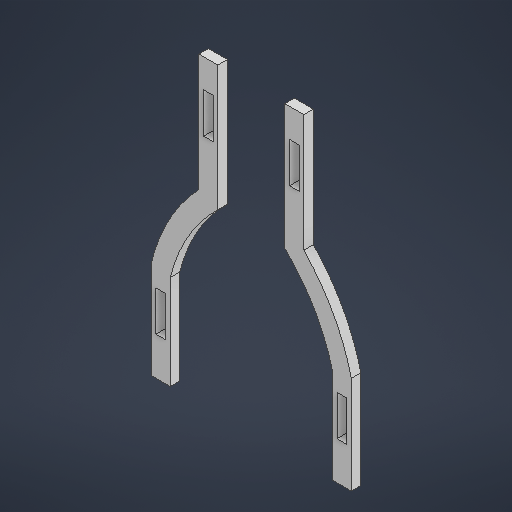
# Autodesk Inventor part: middlelsidewall
Saved by Autodesk Inventor 2026.2 (Build 302298000, 298)
## iProperties
Created: 2026-04-17
Part Number: middlelsidewall
Material: Generic
Document SubType Name: Modeling
Designer: danda
Density: 1 g/cm^3
Appearance: Default
Author: danda
Autodesk Inventor part; units mm, degrees
ref_plane "YZ Plane" through (0, 0, 0) normal (1, 0, 0) x (0, 1, 0)
ref_plane "XZ Plane" through (0, 0, 0) normal (0, 1, 0) x (-1, 0, 0)
ref_plane "XY Plane" through (0, 0, 0) normal (0, 0, 1) x (1, 0, 0)
sketch "Sketch2" plane through (0, 0, 0) normal (0, 0, 1) x (1, 0, 0)
  line L0 (32.8823, 96.9088) -> (32.8823, 36.9088)
  line L1 (-2.1177, 96.9088) -> (-2.1177, 36.9088)
  arc A0 (-2.1177, 36.9088) -> (-27.1177, -6.3925) centre (60.2572, -27.9709) ccw
  line L2 (-2.1177, 36.9088) -> (-27.1177, -6.3925) construction
  line L3 (-2.1177, 36.9088) -> (47.8823, 36.9088) construction
  line L4 (-27.1177, -6.3925) -> (-27.1177, -56.3925)
  arc A1 (57.7441, -5.8406) -> (32.8823, 36.9088) centre (-29.4926, -27.9709) ccw
  line L5 (57.7441, -5.8406) -> (57.7441, -55.78)
  line L6 (7.8823, -56.3925) -> (7.8823, -11.1819)
  arc A2 (15.3823, 3.8291) -> (7.8823, -11.1819) centre (60.2572, -27.9709) ccw
  arc A3 (22.7441, -10.7569) -> (15.3823, 3.8291) centre (-29.4926, -27.9709) ccw
  line L7 (22.7441, -10.7569) -> (22.7441, -55.78)
  line L8 (-37.1177, -55.78) -> (-37.1177, -5.2084)
  arc A4 (-12.1177, 41.0354) -> (-37.1177, -5.2084) centre (60.2572, -27.9709) ccw
  line L9 (-12.1177, 41.0354) -> (-12.1177, 102.5213)
  line L10 (-12.1177, 102.5213) -> (42.8823, 102.5213)
  line L11 (42.8823, 102.5213) -> (42.8823, 41.0354)
  arc A5 (67.7441, -4.6253) -> (42.8823, 41.0354) centre (-29.4926, -27.9709) ccw
  line L12 (67.7441, -4.6253) -> (67.7441, -55.78)
  line L13 (-37.1177, -55.78) -> (67.7441, -55.78)
  line L14 (-2.1177, 96.9088) -> (-2.1177, 102.5213)
  line L15 (32.8823, 96.9088) -> (32.8823, 102.5213)
  line L16 (17.7441, -55.78) -> (17.7441, -20.2363)
  line L17 (12.8823, -20.2363) -> (12.8823, -56.3925)
  line L18 (7.8823, -20.2363) -> (12.8823, -20.2363)
  line L19 (17.7441, -20.2363) -> (22.7441, -20.2363)
  line L20 (32.5233, 96.9088) -> (32.8823, 96.9088)
  line L21 (-2.1177, 67.5213) -> (-2.1177, 87.5213)
  line L22 (32.8823, 67.5213) -> (32.8823, 87.5213)
  line L23 (57.7441, -35.78) -> (57.7441, -15.78)
  line L24 (-27.1177, -15.78) -> (-27.1177, -35.78)
  line L25 (60.2441, -14.78) -> (65.2441, -14.78)
  line L26 (65.2441, -14.78) -> (65.2441, -35.78)
  line L27 (65.2441, -35.78) -> (60.2441, -35.78)
  line L28 (60.2441, -35.78) -> (60.2441, -14.78)
  line L29 (-34.5956, -14.78) -> (-29.5956, -14.78)
  line L30 (-29.5956, -14.78) -> (-29.5956, -35.78)
  line L31 (-29.5956, -35.78) -> (-34.5956, -35.78)
  line L32 (-34.5956, -35.78) -> (-34.5956, -14.78)
  line L33 (35.3823, 87.5213) -> (40.3823, 87.5213)
  line L34 (40.3823, 87.5213) -> (40.3823, 66.5213)
  line L35 (40.3823, 66.5213) -> (35.3823, 66.5213)
  line L36 (35.3823, 66.5213) -> (35.3823, 87.5213)
  line L37 (-9.6177, 87.5213) -> (-4.6177, 87.5213)
  line L38 (-4.6177, 87.5213) -> (-4.6177, 66.5213)
  line L39 (-4.6177, 66.5213) -> (-9.6177, 66.5213)
  line L40 (-9.6177, 66.5213) -> (-9.6177, 87.5213)
  point P0 (0, 0)
  point P1 (-18.405, 65.3533)
  point P2 (-27.1177, -55.78)
  dimension "d25" = 35
  dimension "d26" = 60
  dimension "d27" = 50
  dimension "d28" = 120
  dimension "d29" = 90
  dimension "d30" = 50
  dimension "d31" = 35
  dimension "d32" = 10
  dimension "d33" = 5
  dimension "d34" = 10
  dimension "d35" = 158.3013
  dimension "d36" = 0
  dimension "d37" = 5
  dimension "d38" = 21
  dimension "d39" = 5
  dimension "d40" = 21
  dimension "d41" = 5
  dimension "d42" = 21
  dimension "d43" = 5
  dimension "d44" = 21
  dimension "d45" = 2.5
  dimension "d46" = 15
  dimension "d47" = 2.5
  dimension "d48" = 15
  dimension "d49" = 20
  dimension "d50" = 20
  constraints: 82 end point, 13 point on line, 12 point on circle, 9 perpendicular, 8 parallel, 7 horizontal, 6 centre point, 2 vertical, 1 equal length, 5 other
  measures "d25" distance of L1.start L15.start
  measures "d26" distance of L15.start L0.end
  measures "d27" distance of L1.end L2.end
  measures "d28" angle of L2 L3
  measures "d29" radius of A0
  measures "d30" distance of L2.end L4.end
  measures "d31" distance between parallel lines of L4 L6
  measures "d32" distance between parallel lines of L1 L9
  measures "d33" distance between parallel lines of L7 L16
  measures "d34" distance between parallel lines of L11 L0
  measures "d35" distance between parallel lines of L13 L10
  measures "d36" distance between parallel lines of L4 L24
  measures "d37" distance of L26.end L28.start
  measures "d38" distance of L25.end L26.end
  measures "d39" distance of L30.end L32.start
  measures "d40" distance of L30.start L30.end
  measures "d41" distance of L34.end L36.start
  measures "d42" distance of L34.start L34.end
  measures "d43" distance of L38.end L39.end
  measures "d44" distance of L37.end L38.end
  measures "d45" distance between parallel lines of L1 L38
  measures "d46" distance between parallel lines of L10 L37
  measures "d47" distance between parallel lines of L11 L34
  measures "d48" distance between parallel lines of L10 L33
  measures "d49" distance between parallel lines of L13 L31
  measures "d50" distance between parallel lines of L13 L27
extrude "Extrusion2" add sketch "Sketch2" along normal blind 5 contours L15 L10 L11 A5 L12 L13 L5 A1 L0 | L14 L1 A0 L4 L13 L8 A4 L9 L10
equation "\"d34\" = d32"
body "Solid2"
